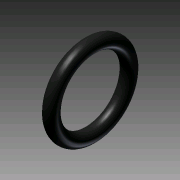
# Autodesk Inventor part: O Ring 1 R.609 1764
Saved by Autodesk Inventor 2011 (Build 150239000, 239)
## iProperties
Created: 2007-11-29
Part Number: O Ring 1 R.609 1764
Document SubType Name: Modeling
Designer: lwoods
Density: 1 g/cm^3
Author: lwoods
Autodesk Inventor part; units mm, degrees
ref_plane "YZ Plane" through (0, 0, 0) normal (1, 0, 0) x (0, 1, 0)
ref_plane "XZ Plane" through (0, 0, 0) normal (0, 1, 0) x (-1, 0, 0)
ref_plane "XY Plane" through (0, 0, 0) normal (0, 0, 1) x (1, 0, 0)
sketch "Sketch1" plane through (0, 0, 0) normal (0, 0, 1) x (1, 0, 0)
  circle A0 centre (-18.8889, 8.0996) radius 1.5875
  line L0 (-29.2593, -1.2222) -> (-5.1852, -1.2222)
  line L1 (-18.8889, 8.0996) -> (-18.8889, 6.5121)
  line L2 (-18.8889, 6.5121) -> (-18.8889, -1.2222)
  dimension "d0" = 3.175
  dimension "d1" = 7.7343
  constraints: 6 end point, 2 perpendicular, 1 horizontal, 1 point on line, 1 vertical alignment, 2 other
  measures "d1" distance of L1.end L2.end
revolve "Revolution1" add sketch "Sketch1" angle 360 about axis through (-29.2593, -1.2222, 0) along (1, 0, 0)
body "Solid1"
